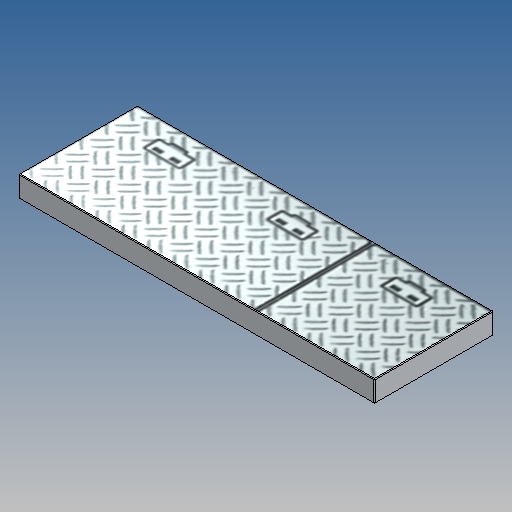
# Autodesk Inventor part: 42146_69729_3
Saved by Autodesk Inventor 2025 (Build 290162010, 162A)
## iProperties
Created: 2021-04-07
Part Number: 42146_69729_3
Material: ABS Plastic
Document SubType Name: Modeling
Designer: D. Kohfeld
Density: 1.06 g/cm^3
Appearance: LtBluishGray
Mass: 1.7301 g
Surface Area: 24.0414 cm^2
Volume: 1.63217 cm^3
Author: D. Kohfeld
Autodesk Inventor part; units mm, degrees
ref_plane "YZ Plane" through (0, 0, 0) normal (1, 0, 0) x (0, 1, 0)
ref_plane "XZ Plane" through (0, 0, 0) normal (0, 1, 0) x (-1, 0, 0)
ref_plane "XY Plane" through (0, 0, 0) normal (0, 0, 1) x (1, 0, 0)
sketch "Sketch2" plane through (0, 0, 0) normal (0, 1, 0) x (-1, 0, 0)
  line L0 (-24, 8) -> (24, 8)
  line L1 (24, 8) -> (24, -8)
  line L2 (24, -8) -> (-24, -8)
  line L3 (-24, -8) -> (-24, 8)
  line L4 (-23.6, 7.6) -> (23.6, 7.6)
  line L5 (23.6, 7.6) -> (23.6, -7.6)
  line L6 (23.6, -7.6) -> (-23.6, -7.6)
  line L7 (-23.6, -7.6) -> (-23.6, 7.6)
  circle A0 centre (0, 0) radius 2.4
  circle A1 centre (0, 0) radius 3.2
  circle A2 centre (-8, 0) radius 2.4
  circle A3 centre (-8, 0) radius 3.2
  circle A4 centre (-16, 0) radius 2.4
  circle A5 centre (-16, 0) radius 3.2
  circle A6 centre (8, 0) radius 2.4
  circle A7 centre (8, 0) radius 3.2
  circle A8 centre (16, 0) radius 2.4
  circle A9 centre (16, 0) radius 3.2
  line L8 (16, 0) -> (8, 0) construction
  line L9 (8, 0) -> (0, 0) construction
  line L10 (0, 0) -> (-8, 0) construction
  line L11 (-8, 0) -> (-16, 0) construction
  line L12 (-22.4, 6.4) -> (22.4, 6.4)
  line L13 (22.4, 6.4) -> (22.4, -6.4)
  line L14 (22.4, -6.4) -> (-22.4, -6.4)
  line L15 (-22.4, -6.4) -> (-22.4, 6.4)
  circle A10 centre (-20, 4) radius 2.4 construction
  circle A11 centre (-20, -4) radius 2.4 construction
  circle A12 centre (20, 4) radius 2.4 construction
  circle A13 centre (20, -4) radius 2.4 construction
  point P0 (0, 8)
  point P1 (-24, 0)
  point P2 (0, 7.6)
  point P3 (-23.6, 0)
  point P4 (0, 6.4)
  point P5 (-22.4, 0)
  dimension "d0" = 16
  dimension "d1" = 48
  dimension "d2" = 0.4
  dimension "d3" = 0.4
  dimension "d4" = 4.8
  dimension "d5" = 6.4
  dimension "d6" = 8
  dimension "d7" = 1.6
  dimension "d8" = 1.6
  dimension "d15" = 4.8
  constraints: 32 end point, 14 centre point, 11 equal radius, 8 tangent, 7 horizontal, 6 coincident, 6 midpoint, 6 parallel, 3 collinear, 3 horizontal alignment, 3 perpendicular, 3 vertical alignment
  measures "d0" distance of L2.end L0.start
  measures "d1" distance of L0.start L0.end
  measures "d2" distance between parallel lines of L0 L4
  measures "d3" distance between parallel lines of L3 L7
  measures "d4" diameter of A0
  measures "d5" diameter of A1
  measures "d6" distance of L9.end L10.end
  measures "d7" distance between parallel lines of L3 L15
  measures "d8" distance between parallel lines of L0 L12
  measures "d15" diameter of A12
extrude "Extrusion1" add sketch "Sketch2" along normal blind 3.2 contours L0 L1 L2 L3 | L4 L5 L6 L7 | A0 | A1 | A2 | A3 | A4 | A5 | A6 | A7 | A8 | A9 | L12 L13 L14 L15
extrude "Extrusion2" cut sketch "Sketch2" along normal blind 0.4 contours L0 L1 L2 L3
extrude "Extrusion3" cut sketch "Sketch2" along normal blind 1.6 contours A0 | A2 | A4 | A6 | A8 | L12 L13 L14 L15
fillet "Fillet1" radius 0.1 8 edges at (-24, 1.8, 8) (0, 3.2, 8) (-24, 3.2, 0) (-24, 1.8, -8) (0, 3.2, -8) (24, 1.8, -8) (24, 3.2, 0) (24, 1.8, 8)
sketch "Skizze3" plane through (0, 3.2, 0) normal (0, 1, 0) x (1, 0, 0)
  line L0 (23.9, 7.9) -> (23.9, -7.9) projected
  line L1 (-23.9, 7.9) -> (23.9, 7.9) projected
  line L2 (-23.9, -7.9) -> (-23.9, 7.9) projected
  line L3 (23.9, -7.9) -> (-23.9, -7.9) projected
  line L4 (-23.9, -8) -> (23.9, -8) projected
  line L5 (-24, 7.9) -> (-24, -7.9) projected
  line L6 (23.9, 8) -> (-23.9, 8) projected
  line L7 (-24.9, -8) -> (-24.9, 8.7) construction
  line L8 (-24.9, 8.7) -> (28.8414, 8.7) construction
  line L9 (28.8414, 8.7) -> (28.8414, -8) construction
  line L10 (28.8414, -8) -> (-24.9, -8) construction
  dimension "d49" = 0.9
  dimension "d50" = 0.7
  constraints: 1 collinear, 1 horizontal, 2 other
  measures "d49" distance between parallel lines of L5 L7
  measures "d50" distance between parallel lines of L6 L8
decal "Aufkleber1"
equation "\"d0\" = 2 * lu"
equation "\"d1\" = 6 * lu"
equation "\"d2\" = gw"
equation "\"d3\" = gw"
equation "\"d4\" = kd"
equation "\"d6\" = lu"
equation "\"d7\" = wall"
equation "\"d8\" = wall"
equation "\"d15\" = kd"
equation "\"d9\" = 0.333333 * lh"
equation "\"d11\" = gh"
equation "\"d13\" = 0.333333 * lh - topthk"
equation "\"d16\" = lf"
equation "\"lu\" = 8"
equation "\"gw\" = 0.4"
equation "\"kd\" = 4.8"
equation "\"wall\" = 1.6"
equation "\"lh\" = 9.6"
equation "\"gh\" = 0.4"
equation "\"topthk\" = 1.6"
equation "\"lf\" = 0.1"
body "Solid1"
